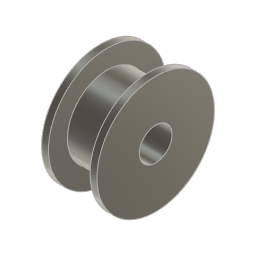
Tensioner (Autodesk Fusion 360 archive; units mm, degrees)
design "20t_pulley"
Autodesk Fusion 360 part; units mm, degrees
sketch "Sketch1" plane through (0, 0, 0) normal (0, 1, 0) x (1, 0, 0)
  line L0 (0, 0) -> (0, -5) construction
  line L1 (0, -2.5) -> (4.225, -2.5)
  line L2 (4.225, -2.5) -> (4.225, -8.96)
  line L3 (4.225, -8.96) -> (3.175, -8.96)
  line L4 (3.175, -8.96) -> (3.175, -6.07)
  line L5 (3.175, -6.07) -> (0, -6.07)
  line L6 (-4.225, -8.96) -> (-3.175, -8.96)
  line L7 (-3.175, -8.96) -> (-3.175, -6.07)
  line L8 (-3.175, -6.07) -> (0, -6.07)
  line L9 (0, -2.5) -> (-4.225, -2.5)
  line L10 (-4.225, -2.5) -> (-4.225, -8.96)
  dimension "d1" = 4.225
  dimension "d2" = 1.05
  dimension "d3" = 2.5
  dimension "d4" = 6.07
  dimension "d5" = 8.96
  constraint coincident L0.start origin
  constraint vertical L0
  constraint midpoint L0 L1.start
  constraint perpendicular L0 L1
  constraint perpendicular L1 L2
  constraint perpendicular L2 L3
  constraint perpendicular L3 L4
  constraint coincident L0 L5.end
  constraint perpendicular L0 L5
  constraint symmetric L0 L1.start L9.start
  constraint symmetric L0 L1.end L9.end
  constraint symmetric L0 L2.end L6.start
  constraint symmetric L0 L3.end L6.end
  constraint symmetric L0 L4.end L7.end
  constraint symmetric L0 L5.end L8.end
  measures "d1" distance of L0 L2
  measures "d2" distance of L2 L4
  measures "d3" distance of L0.start L1
  measures "d4" distance of L0.start L5
  measures "d5" distance of L0.start L3
revolve "Revolve1" add sketch "Sketch1" angle 360 about axis through (1.75, 0, 0) along (1, 0, 0)
ref_plane "WorkPlane1" through (0, 0, 0) normal (-1, 0, 0) x (0, 0, 1)
sketch "Sketch2" plane through (0, 0, 0) normal (-1, 0, 0) x (0, 1, 0)
equation "d1 = ( 8.45 / 2 ) * 1 mm"
equation "d5 = ( 17.92 / 2 ) * 1 mm"
